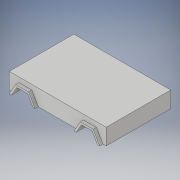
# Autodesk Inventor part: tesla v2
Saved by Autodesk Inventor 2018 (Build 220112000, 112)
## iProperties
Created: 2020-01-07
Part Number: tesla v2
Material: Generic
Document SubType Name: Modeling
Designer: AOFUser
Density: 1 g/cm^3
Appearance: Default
Author: AOFUser
Autodesk Inventor part; units mm, degrees
ref_plane "YZ Plane" through (0, 0, 0) normal (1, 0, 0) x (0, 1, 0)
ref_plane "XZ Plane" through (0, 0, 0) normal (0, 1, 0) x (-1, 0, 0)
ref_plane "XY Plane" through (0, 0, 0) normal (0, 0, 1) x (1, 0, 0)
sketch "Sketch1" plane through (0, 0, 0) normal (0, 1, 0) x (-1, 0, 0)
  line L0 (0, 0) -> (-76.2, 0)
  line L1 (-76.2, 0) -> (-76.2, -50.8)
  line L2 (-76.2, -50.8) -> (0, -50.8)
  line L3 (0, -50.8) -> (0, 0)
  dimension "d0" = 76.2
  dimension "d1" = 50.8
  constraints: 8 end point, 2 parallel, 1 horizontal, 1 perpendicular
  measures "d0" distance of L2.end L1.end
  measures "d1" distance of L1.end L0.end
extrude "Extrusion1" add sketch "Sketch1" along normal blind 12.7
sketch "Sketch5" plane through (76.2, 0, -50.8) normal (0, 0, -1) x (-1, 0, 0)
  line L0 (76.2, 0) -> (73.66, 0)
  line L1 (76.2, 0) -> (0, 0) projected
  line L2 (73.66, 0) -> (53.34, 0)
  line L3 (53.34, 0) -> (58.42, 8.7988)
  line L4 (58.42, 8.7988) -> (68.58, 8.7988)
  line L5 (68.58, 8.7988) -> (73.66, 0)
  dimension "d9" = 2.54
  dimension "d10" = 20.32
  dimension "d11" = 10.16
  dimension "d12" = 60
  dimension "d13" = 10.16
  constraints: 10 end point, 2 point on line, 1 parallel
  measures "d9" distance of L0.start L0.end
  measures "d10" distance of L0.end L2.end
  measures "d11" distance of L2.end L3.end
  measures "d12" angle of L2 L3
  measures "d13" distance of L3.end L4.end
extrude "Extrusion2" add sketch "Sketch5" along normal blind 2.54
sketch "Sketch6" plane through (76.2, 12.7, -50.8) normal (0, 0, -1) x (-1, 0, 0)
  line L0 (76.2, -12.7) -> (0, -12.7) projected
  line L1 (0, -12.7) -> (2.54, -12.7)
  line L2 (2.54, -12.7) -> (22.86, -12.7)
  line L3 (22.86, -12.7) -> (17.78, -3.9012)
  line L4 (17.78, -3.9012) -> (7.62, -3.9012)
  line L5 (7.62, -3.9012) -> (2.54, -12.7)
  dimension "d16" = 2.54
  dimension "d17" = 20.32
  dimension "d18" = 10.16
  dimension "d19" = 60
  dimension "d20" = 10.16
  constraints: 10 end point, 2 point on line, 1 parallel
  measures "d16" distance of L0.end L1.end
  measures "d17" distance of L1.end L2.end
  measures "d18" distance of L2.end L3.end
  measures "d19" angle of L3 L2
  measures "d20" distance of L3.end L4.end
extrude "Extrusion3" add sketch "Sketch6" along normal blind 2.54
sketch "Sketch7" plane through (0, 0, 0) normal (0, 0, 1) x (1, 0, 0)
  line L0 (2.54, 0) -> (0, 0) projected
  line L1 (0, 0) -> (2.54, 0)
  line L2 (22.86, 0) -> (2.54, 0) projected
  line L3 (2.54, 0) -> (22.86, 0)
  line L4 (22.86, 0) -> (17.78, 8.7988) projected
  line L5 (22.86, 0) -> (17.78, 8.7988)
  line L6 (17.78, 8.7988) -> (7.62, 8.7988) projected
  line L7 (17.78, 8.7988) -> (7.62, 8.7988)
  line L8 (7.62, 8.7988) -> (2.54, 0) projected
  line L9 (7.62, 8.7988) -> (2.54, 0)
  dimension "d23" = 20.32
  dimension "d24" = 10.16
  dimension "d25" = 60
  constraints: 10 end point, 4 collinear, 1 horizontal
  measures "d23" distance of L0.start L2.start
  measures "d24" distance of L2.start L4.end
  measures "d25" angle of L5 L3
extrude "Extrusion4" add sketch "Sketch7" along normal blind 2.54
sketch "Sketch8" plane through (0, 12.7, 0) normal (0, 0, 1) x (1, 0, 0)
  line L0 (76.2, -12.7) -> (73.66, -12.7) projected
  line L1 (76.2, -12.7) -> (73.66, -12.7)
  line L2 (53.34, -12.7) -> (58.42, -3.9012) projected
  line L3 (73.66, -12.7) -> (53.34, -12.7)
  line L4 (53.34, -12.7) -> (58.42, -3.9012)
  line L5 (58.42, -3.9012) -> (68.58, -3.9012)
  line L6 (68.58, -3.9012) -> (73.66, -12.7) projected
  line L7 (68.58, -3.9012) -> (73.66, -12.7)
  point P0 (0, -12.7)
  dimension "d28" = 10.16
  constraints: 10 end point, 4 collinear, 1 parallel
  measures "d28" distance of L2.end L5.end
extrude "Extrusion5" add sketch "Sketch8" along normal blind 2.54
sketch "Sketch10" plane through (76.2, 12.7, -53.34) normal (0, 0, -1) x (-1, 0, 0)
  line L0 (7.62, -3.9012) -> (2.54, -12.7) projected
  line L1 (2.54, -12.7) -> (12.7, -12.7)
  line L2 (2.54, -12.7) -> (22.86, -12.7) projected
  line L3 (2.54, -12.7) -> (4.318, -12.7)
  line L4 (4.318, -12.7) -> (8.509, -5.441)
  line L5 (8.509, -5.441) -> (16.891, -5.441)
  line L6 (16.891, -5.441) -> (21.082, -12.7)
  line L7 (21.082, -12.7) -> (16.891, -19.959)
  line L8 (16.891, -19.959) -> (8.509, -19.959)
  line L9 (8.509, -19.959) -> (4.318, -12.7)
  point P0 (76.2, -12.7)
  dimension "d31" = 1.778
  constraints: 16 end point, 1 coincident, 1 midpoint, 1 point on line, 13 other
  measures "d31" distance of L0.end L3.end
extrude "Extrusion6" cut sketch "Sketch10" against normal blind 7.62
sketch "Sketch11" plane through (76.2, 0, -53.34) normal (0, 0, -1) x (-1, 0, 0)
  line L0 (53.34, 0) -> (73.66, 0) projected
  line L1 (53.34, 0) -> (63.5, 0)
  line L2 (22.86, 0) -> (53.34, 0) projected
  line L3 (53.34, 0) -> (55.118, 0)
  line L4 (55.118, 0) -> (59.309, 7.259)
  line L5 (59.309, 7.259) -> (67.691, 7.259)
  line L6 (67.691, 7.259) -> (71.882, 0)
  line L7 (71.882, 0) -> (67.691, -7.259)
  line L8 (67.691, -7.259) -> (59.309, -7.259)
  line L9 (59.309, -7.259) -> (55.118, 0)
  point P0 (76.2, 0)
  dimension "d34" = 10.16
  dimension "d35" = 1.778
  constraints: 16 end point, 1 coincident, 1 midpoint, 1 point on line, 13 other
  measures "d34" distance of L0.start L1.end
  measures "d35" distance of L0.start L3.end
extrude "Extrusion7" cut sketch "Sketch11" against normal blind 7.62
sketch "Sketch12" plane through (0, 0, 2.54) normal (0, 0, 1) x (1, 0, 0)
  line L0 (0, 0) -> (2.54, 0) projected
  line L1 (2.54, 0) -> (12.7, 0)
  line L2 (2.54, 0) -> (22.86, 0) projected
  line L3 (2.54, 0) -> (4.318, 0)
  line L4 (4.318, 0) -> (8.509, 7.259)
  line L5 (8.509, 7.259) -> (16.891, 7.259)
  line L6 (16.891, 7.259) -> (21.082, 0)
  line L7 (21.082, 0) -> (16.891, -7.259)
  line L8 (16.891, -7.259) -> (8.509, -7.259)
  line L9 (8.509, -7.259) -> (4.318, 0)
  dimension "d38" = 10.16
  dimension "d39" = 1.778
  constraints: 16 end point, 1 coincident, 1 midpoint, 1 point on line, 13 other
  measures "d38" distance of L0.end L1.end
  measures "d39" distance of L0.end L3.end
extrude "Extrusion8" cut sketch "Sketch12" against normal blind 7.62
sketch "Sketch13" plane through (0, 12.7, 2.54) normal (0, 0, 1) x (1, 0, 0)
  line L0 (22.86, -12.7) -> (53.34, -12.7) projected
  line L1 (53.34, -12.7) -> (63.5, -12.7)
  line L2 (53.34, -12.7) -> (73.66, -12.7) projected
  line L3 (53.34, -12.7) -> (55.118, -12.7)
  line L4 (55.118, -12.7) -> (59.309, -5.441)
  line L5 (59.309, -5.441) -> (67.691, -5.441)
  line L6 (67.691, -5.441) -> (71.882, -12.7)
  line L7 (71.882, -12.7) -> (67.691, -19.959)
  line L8 (67.691, -19.959) -> (59.309, -19.959)
  line L9 (59.309, -19.959) -> (55.118, -12.7)
  point P0 (0, -12.7)
  dimension "d42" = 10.16
  dimension "d43" = 1.778
  constraints: 16 end point, 1 coincident, 1 midpoint, 1 point on line, 13 other
  measures "d42" distance of L0.end L1.end
  measures "d43" distance of L0.end L3.end
extrude "Extrusion9" cut sketch "Sketch13" against normal blind 7.62
body "Solid1"
